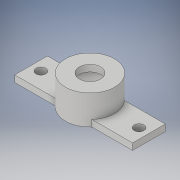
# Autodesk Inventor part: LED_mount2
Saved by Autodesk Inventor 2019 (Build 230136000, 136)
## iProperties
Created: 2018-10-08
Part Number: LED_mount2
Material: Generic
Document SubType Name: Modeling
Designer: Misha
Density: 1 g/cm^3
Appearance: Default
Author: Misha
Autodesk Inventor part; units mm, degrees
ref_plane "YZ Plane" through (0, 0, 0) normal (1, 0, 0) x (0, 1, 0)
ref_plane "XZ Plane" through (0, 0, 0) normal (0, 1, 0) x (-1, 0, 0)
ref_plane "XY Plane" through (0, 0, 0) normal (0, 0, 1) x (1, 0, 0)
sketch "Sketch1" plane through (0, 0, 0) normal (0, 1, 0) x (-1, 0, 0)
  line L0 (0, 0) -> (0, -10)
  line L1 (0, -10) -> (36, -10)
  line L2 (36, -10) -> (36, 0)
  line L3 (36, 0) -> (0, 0)
  circle A0 centre (33, -5) radius 1.5
  circle A1 centre (3, -5) radius 1.5
  dimension "d0" = 10
  dimension "d1" = 36
  constraints: 8 end point, 3 perpendicular, 2 centre point, 1 vertical
  measures "d0" distance of L0.start L0.end
  measures "d1" distance of L0.end L1.end
extrude "Extrusion1" add sketch "Sketch1" along normal blind 2
sketch "Sketch2" plane through (0, 2, 0) normal (0, 1, 0) x (1, 0, 0)
  line L0 (-36, 0) -> (0, 0) projected
  line L1 (-18, 0) -> (-18, 10)
  line L2 (0, 10) -> (-36, 10) projected
  circle A0 centre (-18, 5) radius 7.5
  dimension "d6" = 15
  constraints: 3 midpoint, 2 end point, 1 centre point
  measures "d6" diameter of A0
extrude "Extrusion2" add sketch "Sketch2" along normal blind 7
sketch "Sketch5" plane through (0, 2, 0) normal (0, -1, 0) x (1, 0, 0)
  arc A0 (-13.4654, 0) -> (-22.5346, 0) centre (-18, -5) ccw projected
  circle A1 centre (-18, -5) radius 7.5
  point P0 (0, 0)
  constraints: 1 centre point, 1 coincident
extrude "Extrusion5" add sketch "Sketch5" along normal blind 2
sketch "Sketch8" plane through (-18, 9, -5) normal (0, 1, 0) x (1, 0, 0)
  circle A0 centre (0, 0) radius 3.25
  point P0 (18, -5)
  dimension "d19" = 6.5
  constraints: 1 centre point
  measures "d19" diameter of A0
extrude "Extrusion7" cut sketch "Sketch8" against normal up to next
sketch "Sketch9" plane through (0, 0, 0) normal (0, -1, 0) x (1, 0, 0)
  circle A0 centre (-18, -5) radius 3.25 projected
  circle A1 centre (-18, -5) radius 6.75
  point P0 (0, 0)
  dimension "d22" = 13.5
  constraints: 1 centre point, 1 coincident
  measures "d22" diameter of A1
extrude "Extrusion8" cut sketch "Sketch9" against normal blind 7
body "Solid1"
